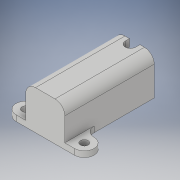
# Autodesk Inventor part: 14 slot pinhuls groot
Saved by Autodesk Inventor 2019 (Build 230136000, 136)
## iProperties
Created: 2021-01-12
Part Number: 14 slot pinhuls groot
Material: Generic
Document SubType Name: Modeling
Designer: semboonen
Density: 1 g/cm^3
Appearance: Default
Author: semboonen
Autodesk Inventor part; units mm, degrees
ref_plane "YZ Plane" through (0, 0, 0) normal (1, 0, 0) x (0, 1, 0)
ref_plane "XZ Plane" through (0, 0, 0) normal (0, 1, 0) x (-1, 0, 0)
ref_plane "XY Plane" through (0, 0, 0) normal (0, 0, 1) x (1, 0, 0)
sketch "Sketch1" plane through (0, 0, 0) normal (0, 0, 1) x (1, 0, 0)
  line L0 (-6.25, 6.25) -> (6.25, 6.25)
  line L1 (6.25, 6.25) -> (6.25, -6.25)
  line L2 (6.25, -6.25) -> (-6.25, -6.25)
  line L3 (-6.25, -6.25) -> (-6.25, 6.25)
  line L4 (-10, 10) -> (10, 10)
  line L5 (10, 10) -> (10, -10)
  line L6 (10, -10) -> (-10, -10)
  line L7 (-10, -10) -> (-10, 10)
  line L8 (-10, 10) -> (10, -10) construction
  line L9 (10, 10) -> (-10, -10) construction
  dimension "d3" = 20
  dimension "d4" = 20
  dimension "d5" = 3.75
  dimension "d6" = 16.25
  dimension "d7" = 3.75
  dimension "d8" = 16.25
  constraints: 20 end point, 5 parallel, 2 perpendicular, 1 horizontal
  measures "d3" distance of L5.end L6.end
  measures "d4" distance of L4.end L5.end
  measures "d5" distance between parallel lines of L1 L5
  measures "d6" distance between parallel lines of L3 L5
  measures "d7" distance between parallel lines of L0 L4
  measures "d8" distance between parallel lines of L2 L4
extrude "Extrusion1" add sketch "Sketch1" along normal blind 55
sketch "Sketch2" plane through (0, 0, 55) normal (0, 0, 1) x (1, 0, 0)
  line L0 (10, 10) -> (-10, 10) projected
  line L1 (-10, -10) -> (10, -10)
  line L2 (10, -10) -> (10, 10)
  line L3 (10, 10) -> (-10, 10)
  line L4 (-10, 10) -> (-10, -10)
  line L5 (-10, -10) -> (10, 10) construction
  line L6 (10, -10) -> (-10, 10) construction
  point P0 (0, 0)
  constraints: 12 end point, 2 midpoint, 2 parallel, 1 horizontal, 1 perpendicular
extrude "Extrusion2" add sketch "Sketch2" along normal blind 3
sketch "Sketch3" plane through (0, 0, 55) normal (0, 0, -1) x (-1, 0, 0)
  circle A0 centre (0, 0) radius 4
  dimension "d13" = 8
  constraints: 1 centre point, 1 coincident
  measures "d13" diameter of A0
extrude "Extrusion3" add sketch "Sketch3" along normal blind 14
sketch "Sketch4" plane through (10, -10, 0) normal (1, 0, 0) x (0, 0, -1)
  line L0 (0, 0) -> (-58, 0) projected
  line L1 (0, 0) -> (-10, 0)
  line L2 (-10, 0) -> (-10, 3)
  line L3 (-10, 3) -> (0, 3)
  line L4 (0, 3) -> (0, 0)
  line L5 (-58, 0) -> (-58, 20) projected
  line L6 (-58, 0) -> (-48, 0)
  line L7 (-48, 0) -> (-48, 3)
  line L8 (-48, 3) -> (-58, 3)
  line L9 (-58, 3) -> (-58, 0)
  point P0 (0, 10)
  dimension "d16" = 10
  dimension "d17" = 3
  dimension "d18" = 10
  dimension "d19" = 3
  constraints: 16 end point, 4 parallel, 2 horizontal, 2 perpendicular
  measures "d16" distance of L2.end L3.end
  measures "d17" distance of L1.end L2.end
  measures "d18" distance of L8.end L7.end
  measures "d19" distance of L7.end L6.end
extrude "Extrusion4" add sketch "Sketch4" along normal blind 10
sketch "Sketch5" plane through (-10, -10, 0) normal (-1, 0, 0) x (0, 0, 1)
  line L0 (0, 0) -> (0, 20) projected
  line L1 (0, 3) -> (10, 3) projected
  line L2 (0, 0) -> (10, 0)
  line L3 (10, 0) -> (10, 3)
  line L4 (10, 3) -> (0, 3)
  line L5 (0, 3) -> (0, 0)
  line L6 (58, 20) -> (58, 0) projected
  line L7 (58, 0) -> (48, 0)
  line L8 (48, 0) -> (48, 3)
  line L9 (48, 3) -> (58, 3)
  line L10 (58, 3) -> (58, 0)
  point P0 (0, 10)
  dimension "d22" = 10
  dimension "d23" = 3
  dimension "d24" = 10
  dimension "d25" = 3
  constraints: 16 end point, 4 parallel, 2 horizontal, 2 perpendicular
  measures "d22" distance of L4.end L1.end
  measures "d23" distance of L1.end L2.end
  measures "d24" distance of L8.end L9.end
  measures "d25" distance of L7.end L8.end
extrude "Extrusion5" add sketch "Sketch5" along normal blind 10
fillet "Fillet1" radius 5 12 edges at (-20, -8.5, 10) (-20, -8.5, 0) (-10, -8.5, 10) (-10, -8.5, 48) (-20, -8.5, 48) (-20, -8.5, 58) (20, -8.5, 0) (10, -8.5, 10) (20, -8.5, 10) (10, -8.5, 48) (20, -8.5, 48) (20, -8.5, 58)
sketch "Sketch6" plane through (10, -7, 15) normal (0, 1, 0) x (1, 0, 0)
  arc A0 (-25, 15) -> (-25, 5) centre (-25, 10) ccw projected
  circle A1 centre (-25, 10) radius 2
  arc A2 (5, 5) -> (5, 15) centre (5, 10) ccw projected
  circle A3 centre (5, 10) radius 2
  arc A4 (-25, -33) -> (-25, -43) centre (-25, -38) ccw projected
  circle A5 centre (-25, -38) radius 2
  arc A6 (5, -43) -> (5, -33) centre (5, -38) ccw projected
  circle A7 centre (5, -38) radius 2
  point P0 (-10, 15)
  dimension "d29" = 4
  dimension "d30" = 4
  dimension "d31" = 4
  constraints: 4 centre point, 4 coincident, 1 equal radius
  measures "d29" diameter of A1
  measures "d30" diameter of A3
  measures "d31" diameter of A5
extrude "Extrusion6" cut sketch "Sketch6" against normal blind 10
fillet "Fillet2" radius 5 2 edges at (-10, 10, 29) (10, 10, 29)
sketch "Sketch7" plane through (-5, 10, 0) normal (0, 1, 0) x (1, 0, 0)
  arc A0 (7.7, -10) -> (2.3, -10) centre (5, -10) ccw
  line L0 (0, -58) -> (0, 0) projected
  arc A1 (2.3, -14.35) -> (7.7, -14.35) centre (5, -14.35) ccw
  line L1 (2.3, -14.35) -> (2.3, -10)
  line L2 (7.7, -14.35) -> (7.7, -10)
  point P0 (5, 0)
  dimension "d35" = 5.4
  dimension "d36" = 5
  dimension "d37" = 10
  dimension "d38" = 5.4
  dimension "d39" = 4.35
  dimension "d40" = 5
  constraints: 4 end point, 4 point on circle, 4 tangent, 2 centre point
  measures "d35" diameter of A0
  measures "d36" distance from line of L0 A0.centre
  measures "d37" distance of point (5, 0) A0.centre
  measures "d38" diameter of A1
  measures "d39" distance of A1.centre A0.centre
  measures "d40" distance from line of L0 A1.centre
extrude "Extrusion7" cut sketch "Sketch7" against normal blind 10
sketch "Sketch8" plane through (-5, 10, 0) normal (0, 1, 0) x (1, 0, 0)
  line L0 (2.3, -10) -> (2.3, -14.35) projected
  line L1 (2.3, -12.175) -> (-5, -12.175)
  line L2 (-5, 0) -> (-5, -58) projected
  arc A0 (-5, -15) -> (-10, -10) centre (-10, -15) ccw projected
  line L3 (-5, -12.175) -> (-5, -15)
  line L4 (-5, -15) -> (-18.139, -15)
  line L5 (-18.139, -15) -> (-18.139, 3.699)
  line L6 (-18.139, 3.699) -> (27.6458, 3.699)
  line L7 (27.6458, 3.699) -> (27.6458, -15)
  line L8 (15, -15) -> (15, -43) projected
  line L9 (27.6458, -15) -> (15, -15)
  line L10 (15, -15) -> (15, -12.175)
  arc A1 (20, -10) -> (15, -15) centre (20, -15) ccw projected
  line L11 (15, -12.175) -> (2.3, -12.175)
  point P0 (5, 0)
  dimension "d43" = 12.6458
  dimension "d44" = 33.139
  dimension "d45" = 18.699
  constraints: 18 end point, 7 perpendicular, 3 point on line, 2 tangent, 1 horizontal, 1 midpoint, 1 vertical
  measures "d43" distance between parallel lines of L7 L8
  measures "d44" distance between parallel lines of L5 L8
  measures "d45" distance between parallel lines of L6 L9
extrude "Extrusion8" cut sketch "Sketch8" against normal blind 20
sketch "Sketch9" plane through (-2.7, 10, 12.175) normal (0, 0, -1) x (-1, 0, 0)
  circle A0 centre (-10.825, -10) radius 0.925
  circle A1 centre (-2.7, -18.125) radius 0.925
  circle A2 centre (5.425, -10) radius 0.925
  line L0 (-12.7, -20) -> (-12.7, -5) projected
  line L1 (7.3, -20) -> (-12.7, -20) projected
  line L2 (3.55, -16.25) -> (3.55, -3.75) projected
  point P0 (-2.7, -10)
  dimension "d48" = 1.85
  dimension "d49" = 1.85
  dimension "d50" = 1.85
  dimension "d51" = 1.875
  dimension "d52" = 1.875
  dimension "d53" = 1.875
  dimension "d54" = 0
  dimension "d55" = 0
  dimension "d56" = 0
  constraints: 3 centre point
  measures "d48" diameter of A0
  measures "d49" diameter of A1
  measures "d50" diameter of A2
  measures "d51" distance from line of L0 A0.centre
  measures "d52" distance from line of L1 A1.centre
  measures "d53" distance from line of L2 A2.centre
  measures "d54" vertical distance of point (-2.7, -10) A2.centre
  measures "d55" vertical distance of point (-2.7, -10) A0.centre
  measures "d56" horizontal distance of point (-2.7, -10) A1.centre
extrude "Extrusion9" cut sketch "Sketch9" against normal blind 5
body "Solid1"
